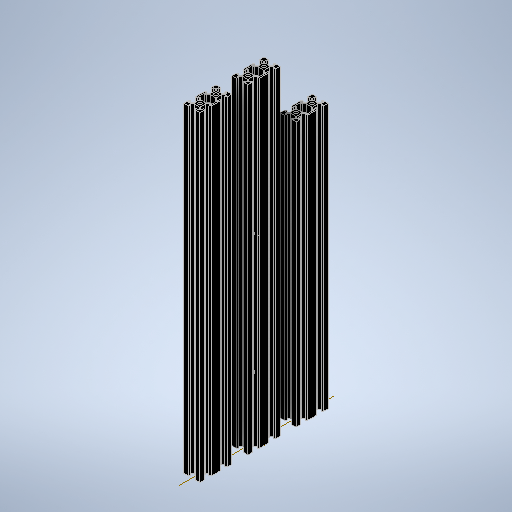
# Autodesk Inventor part: 2040 Extrusions
Saved by Autodesk Inventor 2025 (Build 290162000, 162)
## iProperties
Created: 2025-02-05
Part Number: 2040 Extrusions
Material: Aluminum 6061
Document SubType Name: Modeling
Designer: MAL16204
Density: 2.7 g/cm^3
Appearance: Anodized - Black
Mass: 162.602 g
Surface Area: 597.082 cm^2
Volume: 60.2229 cm^3
Author: MAL16204
Autodesk Inventor part; units mm, degrees
sketch "Sketch1" plane through (0, 0, 0) normal (0, 1, 0) x (-1, 0, 0)
  circle A0 centre (0, -10) radius 2.1
  circle A1 centre (0, 10) radius 2.1
  line L0 (0, -10) -> (0, 10) construction
  line L1 (3.1, 14.1607) -> (-3.1, 14.1607)
  line L2 (4.1607, 13.1) -> (4.1607, 6.9)
  line L3 (-4.1607, 13.1) -> (-4.1607, 6.9)
  line L4 (0, -67.72) -> (0, 34.62) construction
  line L5 (3.1, -14.1607) -> (-3.1, -14.1607)
  line L6 (-4.1607, -13.1) -> (-4.1607, -6.9)
  line L7 (4.1607, -13.1) -> (4.1607, -6.9)
  line L8 (4.1607, 13.1) -> (6.5607, 15.5)
  line L9 (3.1, 14.1607) -> (5.5, 16.5607)
  line L10 (-3.1, 14.1607) -> (-5.5, 16.5607)
  line L11 (-4.1607, 13.1) -> (-6.5607, 15.5)
  line L12 (3.1, 5.8393) -> (-3.1, 5.8393)
  line L13 (3.1, -5.8393) -> (-3.1, -5.8393)
  line L14 (4.1607, 6.9) -> (6.5607, 4.5)
  line L15 (3.1, 5.8393) -> (5.5, 3.4393)
  line L16 (-3.1, 5.8393) -> (-5.5, 3.4393)
  line L17 (-4.1607, 6.9) -> (-6.5607, 4.5)
  line L18 (4.1607, -13.1) -> (6.5607, -15.5)
  line L19 (3.1, -14.1607) -> (5.5, -16.5607)
  line L20 (-3.1, -14.1607) -> (-5.5, -16.5607)
  line L21 (-4.1607, -13.1) -> (-6.5607, -15.5)
  line L22 (4.1607, -6.9) -> (6.5607, -4.5)
  line L23 (3.1, -5.8393) -> (5.5, -3.4393)
  line L24 (-3.1, -5.8393) -> (-5.5, -3.4393)
  line L25 (-4.1607, -6.9) -> (-6.5607, -4.5)
  line L26 (6.5607, 15.5) -> (8.2, 15.5)
  line L27 (6.5607, 4.5) -> (8.2, 4.5)
  line L28 (-6.5607, 4.5) -> (-8.2, 4.5)
  line L29 (-5.5, 3.4393) -> (-8.2, 3.4393)
  line L30 (-6.5607, 15.5) -> (-8.2, 15.5)
  line L31 (-5.5, 16.5607) -> (-5.5, 18.2)
  line L32 (5.5, 16.5607) -> (5.5, 18.2)
  line L33 (5.5, 3.4393) -> (8.2, 3.4393)
  line L34 (5.5, -16.5607) -> (5.5, -18.2)
  line L35 (-5.5, -16.5607) -> (-5.5, -18.2)
  line L36 (-6.5607, -15.5) -> (-8.2, -15.5)
  line L37 (-6.5607, -4.5) -> (-8.2, -4.5)
  line L38 (6.5607, -15.5) -> (8.2, -15.5)
  line L39 (6.5607, -4.5) -> (8.2, -4.5)
  line L40 (5.5, -3.4393) -> (8.2, -3.4393)
  line L41 (-5.5, -3.4393) -> (-8.2, -3.4393)
  line L42 (5.5, -18.2) -> (3.1, -18.2)
  line L43 (-5.5, -18.2) -> (-3.1, -18.2)
  line L44 (8.2, -15.5) -> (8.2, -13.1)
  line L45 (8.2, -4.5) -> (8.2, -6.9)
  line L46 (-8.2, -4.5) -> (-8.2, -6.9)
  line L47 (-8.2, -15.5) -> (-8.2, -13.1)
  line L48 (8.2, 4.5) -> (8.2, 6.9)
  line L49 (8.2, 15.5) -> (8.2, 13.1)
  line L50 (-8.2, 4.5) -> (-8.2, 6.9)
  line L51 (-8.2, 15.5) -> (-8.2, 13.1)
  line L52 (-5.5, 18.2) -> (-3.1, 18.2)
  line L53 (5.5, 18.2) -> (3.1, 18.2)
  line L54 (8.2, -3.4393) -> (8.2, 3.4393)
  line L55 (-8.2, -3.4393) -> (-8.2, 3.4393)
  line L56 (-3.1, 18.2) -> (-4.775, 20)
  line L57 (3.1, 18.2) -> (4.775, 20)
  line L58 (8.2, 13.1) -> (10, 14.775)
  line L59 (8.2, 6.9) -> (10, 5.225)
  line L60 (-8.2, 6.9) -> (-10, 5.225)
  line L61 (-8.2, 13.1) -> (-10, 14.775)
  line L62 (-8.2, -6.9) -> (-10, -5.225)
  line L63 (-8.2, -13.1) -> (-10, -14.775)
  line L64 (-3.1, -18.2) -> (-4.775, -20)
  line L65 (3.1, -18.2) -> (4.775, -20)
  line L66 (8.2, -13.1) -> (10, -14.775)
  line L67 (8.2, -6.9) -> (10, -5.225)
  line L68 (10, -5.225) -> (10, 5.225)
  line L69 (-10, -5.225) -> (-10, 5.225)
  line L70 (10, 14.775) -> (10, 20)
  line L71 (10, 20) -> (4.775, 20)
  line L72 (-4.775, 20) -> (-10, 20)
  line L73 (-10, 20) -> (-10, 14.775)
  line L74 (10, -14.775) -> (10, -20)
  line L75 (10, -20) -> (4.775, -20)
  line L76 (-4.775, -20) -> (-10, -20)
  line L77 (-10, -20) -> (-10, -14.775)
  line L78 (14, 0) -> (-14, 0) construction
  line L79 (8.2, -13.1) -> (8.2, -6.9) construction
  line L80 (-8.2, -13.1) -> (-8.2, -6.9) construction
  line L81 (3.1, -18.2) -> (-3.1, -18.2) construction
  line L82 (8.2, 13.1) -> (8.2, 6.9) construction
  line L83 (-8.2, 6.9) -> (-8.2, 13.1) construction
  line L84 (-3.1, 18.2) -> (3.1, 18.2) construction
  line L85 (4.1607, 10) -> (-4.1607, 10) construction
  point P0 (0, 0)
  point P1 (0, 0)
  point P2 (0, 14.1607)
  point P3 (0, -14.1607)
  point P4 (0, 5.8393)
  point P5 (0, -5.8393)
  point P6 (10, 0)
  point P7 (-10, 0)
  dimension "d1" = 4.2
  dimension "d8" = 1.8
  dimension "d9" = 1.8
  dimension "d11" = 20
  dimension "d14" = 1.5
  dimension "d15" = 6.2
  dimension "d16" = 40
  dimension "d17" = 9.55
  dimension "d18" = 11
  constraints: 168 end point, 62 equal length, 27 collinear, 24 vertical, 22 horizontal, 10 midpoint, 9 parallel, 5 perpendicular, 2 centre point, 1 coincident, 1 equal radius, 1 point on line, 7 other
  measures "d1" diameter of A1
  measures "d8" distance between parallel lines of L69 L55
  measures "d9" distance between parallel lines of L76 L43
  measures "d11" distance between parallel lines of L73 L70
  measures "d14" distance between parallel lines of L19 L18
  measures "d15" distance of L42.end L43.end
  measures "d16" distance between parallel lines of L71 L75
  measures "d17" distance of L64.end L65.end
  measures "d18" distance between parallel lines of L31 L32
extrude "Extrusion1" add sketch "Sketch1" along normal blind 400
extrude "Extrusion2" add sketch "Sketch1" along normal blind 400 separate body
extrude "Extrusion3" add sketch "Sketch1" along normal blind 330 separate body
move or copy body "Move Body1" bodies to move or copy 2 copy no translate (0, 0, 60)
move or copy body "Move Body2" bodies to move or copy 3 copy no translate (0, 0, -60)
ref_plane "Work Plane1" through (9.1, 0, 5.225) normal (1, 0, 0) x (0, 0, -1)
sketch "Sketch2" plane through (9.1, 0, 5.225) normal (1, 0, 0) x (0, 0, -1)
  line L0 (-47.875, 400) -> (-41.675, 400) projected
  line L1 (-44.775, 400) -> (-44.775, 342.409) construction
  point P0 (5.225, 0)
  point P1 (-44.775, 360.25)
  point P2 (-64.775, 360.25)
  dimension "d32" = 20
  dimension "d33" = 39.75
  constraints: 2 end point, 1 horizontal alignment, 1 midpoint, 1 point on line, 1 vertical
  measures "d32" distance of point (-44.775, 360.25) point (-64.775, 360.25)
  measures "d33" distance from line of L0 point (-44.775, 360.25)
hole "Hole1" at (9.1, 360.25, 50) at (9.1, 360.25, 70) direction (-1, 0, 0) diameter 3.242 end through all bodies 2 thread size "M4x0.7" class "6H" standard "ISO Metric profile"
ref_plane "Work Plane2" through (10, 0, 5.225) normal (1, 0, 0) x (0, 0, -1)
sketch "Sketch3" plane through (10, 0, 5.225) normal (1, 0, 0) x (0, 0, -1)
  line L0 (-1.675, 400) -> (-7.875, 400) construction
  line L1 (-4.775, 400) -> (-4.775, 0) construction
  line L2 (-1.675, 0) -> (-7.875, 0) construction
  point P0 (5.225, 0)
  point P1 (-4.775, 230)
  point P2 (-4.775, 80)
  dimension "d42" = 170
  dimension "d43" = 320
  constraints: 2 end point, 2 midpoint, 2 point on line
  measures "d42" distance from line of L0 point (-4.775, 230)
  measures "d43" distance from line of L0 point (-4.775, 80)
hole "Hole2" at (10, 230, 10) at (10, 80, 10) direction (-1, 0, 0) diameter 3.6881 end through all counterbore diameter 7.5 counterbore depth 5.8 bodies 1 thread size "M4.5x0.75" class "6H" standard "ISO Metric profile"
sketch "Sketch4" plane through (9.1, 0, 5.225) normal (1, 0, 0) x (0, 0, -1)
  line L0 (52.125, 330) -> (58.325, 330) projected
  line L1 (55.225, 330) -> (55.225, 0)
  line L2 (52.125, 0) -> (58.325, 0) projected
  point P0 (5.225, 0)
  constraints: 2 end point, 2 midpoint
ref_plane "Work Plane3" through (4.1607, 0, -73.1) normal (1, 0, 0) x (0, 0, -1)
sketch "Sketch5" plane through (4.1607, 0, -73.1) normal (1, 0, 0) x (0, 0, -1)
  line L0 (-25.2, 330) -> (-21, 330) construction
  line L1 (-23.1, 330) -> (-23.1, 0) construction
  line L2 (-25.2, 0) -> (-21, 0) construction
  line L3 (-5.2, 330) -> (-1, 330) construction
  line L4 (-3.1, 330) -> (-3.1, 0) construction
  point P0 (-73.1, 0)
  point P1 (-23.1, 326)
  point P2 (-23.1, 317)
  point P3 (-23.1, 305)
  point P4 (-3.1, 326)
  dimension "d52" = 4
  dimension "d53" = 13
  dimension "d54" = 25
  constraints: 4 end point, 4 point on line, 3 midpoint, 1 horizontal alignment, 1 vertical
  measures "d52" distance from line of L0 point (-23.1, 326)
  measures "d53" distance from line of L0 point (-23.1, 317)
  measures "d54" distance from line of L0 point (-23.1, 305)
hole "Hole3" at (4.1607, 326, -70) at (4.1607, 305, -50) at (4.1607, 317, -50) at (4.1607, 326, -50) direction (-1, 0, 0) diameter 3.242 end through all bodies 3 thread size "M4x0.7" class "6H" standard "ANSI Metric M Profile"
sketch "Sketch6" plane through (-3.1, 0, -74.1607) normal (0, 0, -1) x (-1, 0, 0)
  line L0 (-6.2, 0) -> (0, 0) construction
  line L1 (-3.1, 0) -> (-3.1, 330.0709) construction
  line L2 (-6.2, 330) -> (0, 330) construction
  point P0 (-3.1, 0)
  point P1 (-3.1, 220)
  point P2 (-3.1, 200)
  dimension "d62" = 110
  dimension "d63" = 130
  constraints: 2 end point, 2 point on line, 1 midpoint, 1 vertical
  measures "d62" distance from line of L2 point (-3.1, 220)
  measures "d63" distance from line of L2 point (-3.1, 200)
hole "Hole4" at (0, 200, -74.1607) at (0, 220, -74.1607) direction (0, 0, 1) diameter 4.134 end through all bodies 3 thread size "M5x0.8" class "6H" standard "ANSI Metric M Profile"
